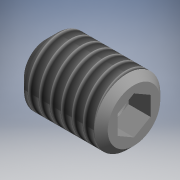
# Autodesk Inventor part: SET-SCREW6-8
Saved by Autodesk Inventor 2017.3 (Build 213256000, 256)
## iProperties
Part Number: SET-SCREW6-8
Material: Generic
Catalog Web Link: www.cadenas.de
Description: SET-SCREW-Set Screw - Flat End
Vendor: MISUMI
Document SubType Name: Modeling
Designer: partserver
Manufacturer: MISUMI
Mass: 0.196883 g
Surface Area: 2.09616 cm^2
Volume: 0.196883 cm^3
Density: 1 g/cm^3
Appearance: PSOLRGB-175-175-175
Category: PARTsolutions
Company: MISUMI
Title: SET-SCREW6-8
Author: Cadenas PARTsolutions
Comments: Set Screw - Flat End
PSOL_IDENT_0: {$CADENAS_DATA\23d-libs\misumi\metric\accessories\set_screw.prj},169 {VTYP=3D},{NB=SET-SCREW6-8},{LI
PSOL_IDENT_1: NA=SET-SCREW6-8},{NN=SET-SCREW},{DATE=30.10.2020 15:47:10},{GEOMDATE=11.12.2013 00:00:00},{VERSION=}
PSOL_IDENT_2: ,{LINEID=70},{WBVAR=L},{WBNUMERIC=L}  {NB=SET-SCREW6-8},{LINA=SET-SCREW6-8},{KT=DUMMY},{PN=SET-SCREW
PSOL_IDENT_3: 6-8},{TYPE=SET-SCREW},{M=6.0},{P=1.00},{L=8},{LMIN=2.9},{LALG=[2.9:42/0.1]},{B=3.0},{C=2.0},{DD=4.0}
NB: SET-SCREW6-8
NN: SET-SCREW
NT: Set Screw - Flat End
NBSYN: $PN.
LINA: SET-SCREW6-8
CATALOG: Misumi
PN: SET-SCREW6-8
M: 6
P: 1
L: 8
B: 3
C: 2
DD: 4
SUPPLIER: MISUMI
ARTICLENO: SET-SCREW6-8
BOMINFO: SET-SCREW6-8
CREATOR: CADENAS GmbH
Autodesk Inventor part; units mm, degrees
sketch "Sketch_1" plane through (0, 0, 0) normal (0, 0, 1) x (1, 0, 0)
  line L0 (0, 0) -> (-8, 0)
  line L1 (-8, 0) -> (-8, 2.3865)
  line L2 (-8, 2.3865) -> (-7.3865, 3)
  line L3 (-7.3865, 3) -> (-1, 3)
  line L4 (-1, 3) -> (0, 2)
  line L5 (0, 2) -> (0, 0)
  line L6 (0, 0) -> (-8, 0)
  constraints: 14 end point
revolve "Revolution1" add sketch "Sketch_1" angle 360 about axis through (0, 0, 0) along (1, 0, 0)
thread "Thread1" size "M6x1" class "6g" standard "ISO Metric profile" full length
sketch "Sketch_2" plane through (-8, 0, 0) normal (-1, 0, 0) x (0, 1, 0)
  line L0 (-1.5, -0.866) -> (0, -1.7321)
  line L1 (0, -1.7321) -> (1.5, -0.866)
  line L2 (1.5, -0.866) -> (1.5, 0.866)
  line L3 (1.5, 0.866) -> (0, 1.7321)
  line L4 (0, 1.7321) -> (-1.5, 0.866)
  line L5 (-1.5, 0.866) -> (-1.5, -0.866)
  constraints: 12 end point
extrude "Extrusion1" cut sketch "Sketch_2" against normal blind 2
sketch "Sketch_3" plane through (0, 0, 0) normal (0, 0, 1) x (1, 0, 0)
  line L0 (-5.134, 0) -> (-6, 0)
  line L1 (-6, 0) -> (-6, 1.5)
  line L2 (-6, 1.5) -> (-5.134, 0)
  line L3 (-5.134, 0) -> (-6, 0)
  constraints: 8 end point
revolve "Revolution2" cut sketch "Sketch_3" angle 360 about axis through (-5.134, 0, 0) along (1, 0, 0)
ref_plane "CP_XY" through (0, 0, 0) normal (1, 0, 0) x (0, 0, -1)
ref_plane "CP_YZ" through (0, 0, 0) normal (0, 0, -1) x (0, 1, 0)
ref_plane "CP_ZX" through (0, 0, 0) normal (0, 1, 0) x (1, 0, 0)
body "Solid1"
